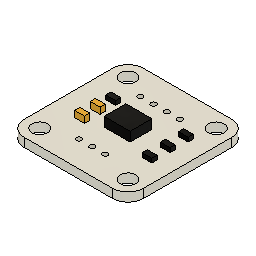
MambaMouse_Rev2 v16 (Autodesk Fusion 360 archive; units mm, degrees)
design "AS5600"
Autodesk Fusion 360 part; units mm, degrees
sketch "Sketch2" plane through (0, 0, 0) normal (0, 1, 0) x (1, 0, 0)
  line L0 (-8.5, -11.5) -> (8.5, -11.5)
  line L1 (11.5, -8.5) -> (11.5, 8.5)
  line L2 (8.5, 11.5) -> (-8.5, 11.5)
  line L3 (-11.5, 8.5) -> (-11.5, -8.5)
  line L4 (-11.5, -11.5) -> (11.5, 11.5) construction
  line L5 (11.5, -11.5) -> (-11.5, 11.5) construction
  line L6 (-8.5, 8.5) -> (8.5, 8.5) construction
  line L7 (8.5, 8.5) -> (8.5, -8.5) construction
  line L8 (8.5, -8.5) -> (-8.5, -8.5) construction
  line L9 (-8.5, -8.5) -> (-8.5, 8.5) construction
  line L10 (-8.5, 8.5) -> (8.5, -8.5) construction
  line L11 (8.5, 8.5) -> (-8.5, -8.5) construction
  circle A0 centre (-8.5, 8.5) radius 1.5
  circle A1 centre (8.5, 8.5) radius 1.5
  circle A2 centre (8.5, -8.5) radius 1.5
  circle A3 centre (-8.5, -8.5) radius 1.5
  arc A4 (-8.5, 11.5) -> (-11.5, 8.5) centre (-8.5, 8.5) ccw
  arc A5 (11.5, 8.5) -> (8.5, 11.5) centre (8.5, 8.5) ccw
  arc A6 (8.5, -11.5) -> (11.5, -8.5) centre (8.5, -8.5) ccw
  arc A7 (-11.5, -8.5) -> (-8.5, -11.5) centre (-8.5, -8.5) ccw
  line L12 (-2.5, -2.1) -> (2.5, -2.1)
  line L13 (2.5, -2.1) -> (2.5, 2.1)
  line L14 (2.5, 2.1) -> (-2.5, 2.1)
  line L15 (-2.5, 2.1) -> (-2.5, -2.1)
  line L16 (-2.5, -2.1) -> (2.5, 2.1) construction
  line L17 (2.5, -2.1) -> (-2.5, 2.1) construction
  circle A8 centre (-4.12, 6.5) radius 0.5
  circle A9 centre (-1.58, 6.5) radius 0.5
  circle A10 centre (0.96, 6.5) radius 0.5
  circle A11 centre (3.5, 6.5) radius 0.5
  line L18 (-4.12, 6.5) -> (-1.58, 6.5) construction
  line L19 (-1.58, 6.5) -> (0.96, 6.5) construction
  line L20 (0.96, 6.5) -> (3.5, 6.5) construction
  circle A12 centre (2.14, -6.5) radius 0.5
  circle A13 centre (-0.4, -6.5) radius 0.5
  circle A14 centre (-2.94, -6.5) radius 0.5
  line L21 (-2.94, -6.5) -> (-0.4, -6.5) construction
  line L22 (-0.4, -6.5) -> (2.14, -6.5) construction
  line L23 (-6.9, 3.63) -> (-5.02, 3.63)
  line L24 (-5.02, 3.63) -> (-5.02, 2.63)
  line L25 (-5.02, 2.63) -> (-6.9, 2.63)
  line L26 (-6.9, 2.63) -> (-6.9, 3.63)
  line L27 (-6.9, 0.63) -> (-5.02, 0.63)
  line L28 (-5.02, 0.63) -> (-5.02, -0.37)
  line L29 (-5.02, -0.37) -> (-6.9, -0.37)
  line L30 (-6.9, -0.37) -> (-6.9, 0.63)
  line L31 (-6.9, -2.37) -> (-5.02, -2.37)
  line L32 (-5.02, -2.37) -> (-5.02, -3.37)
  line L33 (-5.02, -3.37) -> (-6.9, -3.37)
  line L34 (-6.9, -3.37) -> (-6.9, -2.37)
  line L35 (-6.9, 2.63) -> (-6.9, 0.63) construction
  line L36 (-6.9, -0.37) -> (-6.9, -2.37) construction
  line L37 (6.22, 4.5) -> (8.1, 4.5)
  line L38 (8.1, 4.5) -> (8.1, 3.5)
  line L39 (8.1, 3.5) -> (6.22, 3.5)
  line L40 (6.22, 3.5) -> (6.22, 4.5)
  line L41 (6.22, 1) -> (8.1, 1)
  line L42 (8.1, 1) -> (8.1, 0)
  line L43 (8.1, 0) -> (6.22, 0)
  line L44 (6.22, 0) -> (6.22, 1)
  line L45 (6.22, -2.5) -> (8.1, -2.5)
  line L46 (8.1, -2.5) -> (8.1, -3.5)
  line L47 (8.1, -3.5) -> (6.22, -3.5)
  line L48 (6.22, -3.5) -> (6.22, -2.5)
  line L49 (8.1, -2.5) -> (8.1, 0) construction
  line L50 (8.1, 3.5) -> (8.1, 1) construction
  dimension "d6" = 23
  dimension "d7" = 23
  dimension "d8" = 17
  dimension "d9" = 17
  dimension "d10" = 3
  dimension "d11" = 3
  dimension "d12" = 3
  dimension "d13" = 3
  dimension "d14" = 3
  dimension "d15" = 5
  dimension "d16" = 4.2
  dimension "d21" = 1
  dimension "d25" = 2.54
  dimension "d26" = 2.54
  dimension "d27" = 2.54
  dimension "d28" = 5
  dimension "d29" = 8
  dimension "d30" = 2.54
  dimension "d31" = 2.54
  dimension "d32" = 5
  dimension "d33" = 8.56
  dimension "d34" = 1.88
  dimension "d35" = 1
  dimension "d36" = 2
  dimension "d37" = 2
  dimension "d38" = 4.6
  dimension "d39" = 8.13
  dimension "d41" = 3.4
  dimension "d42" = 2.5
  dimension "d43" = 2.5
  dimension "d44" = 8
  constraint horizontal L0
  constraint perpendicular L0 L1
  constraint parallel L0 L2
  constraint parallel L1 L3
  constraint coincident L4 origin
  constraint coincident L5 origin
  constraint horizontal L6
  constraint perpendicular L6 L7
  constraint parallel L6 L8
  constraint parallel L7 L9
  constraint coincident L10 origin
  constraint coincident L11 origin
  constraint coincident L6.start L9.end
  constraint coincident L6.end L7.start
  constraint coincident L7.end L8.start
  constraint coincident L8.end L9.start
  constraint equal A0 A3
  constraint equal A1 A3
  constraint equal A2 A3
  constraint coincident L5.end L3
  constraint coincident L5.end L2
  constraint tangent L3 A4
  constraint tangent L2 A4
  constraint coincident L4.end L2
  constraint coincident L4.end L1
  constraint tangent L2 A5
  constraint tangent L1 A5
  constraint coincident L5.start L0
  constraint coincident L5.start L1
  constraint tangent L0 A6
  constraint tangent L1 A6
  constraint coincident L4.start L3
  constraint coincident L4.start L0
  constraint tangent L3 A7
  constraint tangent L0 A7
  constraint horizontal L12
  constraint perpendicular L12 L13
  constraint parallel L12 L14
  constraint parallel L13 L15
  constraint coincident L16 origin
  constraint coincident L17 origin
  constraint coincident A8.centre L18.start
  constraint coincident A9.centre L18.end
  constraint parallel L6 L18
  constraint coincident A10.centre L19.end
  constraint coincident A11.centre L20.end
  constraint horizontal L19
  constraint horizontal L20
  constraint equal A8 A9
  constraint equal A8 A10
  constraint equal A8 A11
  constraint equal A8 A14
  constraint equal A9 A13
  constraint equal A10 A12
  constraint coincident A14.centre L21.start
  constraint coincident A13.centre L21.end
  constraint horizontal L21
  constraint coincident A12.centre L22.end
  constraint horizontal L22
  constraint horizontal L23
  constraint vertical L24
  constraint horizontal L25
  constraint vertical L26
  constraint horizontal L27
  constraint vertical L28
  constraint horizontal L29
  constraint vertical L30
  constraint horizontal L31
  constraint vertical L32
  constraint horizontal L33
  constraint vertical L34
  constraint equal L23 L27
  constraint equal L27 L31
  constraint equal L24 L28
  constraint equal L28 L32
  constraint vertical L35
  constraint vertical L36
  constraint horizontal L37
  constraint vertical L38
  constraint horizontal L39
  constraint vertical L40
  constraint horizontal L41
  constraint vertical L42
  constraint horizontal L43
  constraint vertical L44
  constraint horizontal L45
  constraint vertical L46
  constraint horizontal L47
  constraint vertical L48
  constraint equal L23 L37
  constraint equal L24 L38
  constraint equal L23 L41
  constraint equal L24 L42
  constraint equal L23 L45
  constraint equal L24 L48
  constraint vertical L50
  constraint vertical L49
  measures "d6" distance of L4.start L5.start
  measures "d7" distance of L5.start L4.end
  measures "d8" distance of L7.end L8.end
  measures "d9" distance of L6.end L7.end
  measures "d10" diameter of A3
  measures "d11" radius of A4
  measures "d12" radius of A5
  measures "d13" radius of A6
  measures "d14" radius of A7
  measures "d15" distance of L13.end L14.end
  measures "d16" distance of L12.end L13.end
  measures "d21" diameter of A8
  measures "d25" distance of A8.centre A9.centre
  measures "d26" horizontal distance of A9.centre A10.centre
  measures "d27" horizontal distance of A10.centre A11.centre
  measures "d28" distance of L2 L18
  measures "d29" distance of L1 A11.centre
  measures "d30" distance of A13.centre A14.centre
  measures "d31" horizontal distance of A12.centre A13.centre
  measures "d32" distance of L0 L22
  measures "d33" distance of L3 A14.centre
  measures "d34" distance of L23.start L23.end
  measures "d35" distance of L23.end L24.end
  measures "d36" distance of L25 L27
  measures "d37" distance of L29 L31
  measures "d38" distance of L3 L35
  measures "d39" distance of L0 L33
  measures "d41" distance of L1 L50
  measures "d42" distance of L38.end L41.end
  measures "d43" distance of L42.end L45.end
  measures "d44" distance of L0 L47
extrude "Extrude1" add sketch "Sketch2" against normal blind 1.7 contours L0 L1 L2 L3 A4 A5 A6 A7 | L12 L13 L14 L15 | L23 L24 L25 L26 | L27 L28 L29 L30 | L31 L32 L33 L34 | L37 L38 L39 L40 | L41 L42 L43 L44 | L45 L46 L47 L48
extrude "Extrude2" add sketch "Sketch2" along normal blind 1.8 contours L12 L13 L14 L15
extrude "Extrude3" add sketch "Sketch2" along normal blind 0.8 contours L23 L24 L25 L26 | L37 L38 L39 L40 | L41 L42 L43 L44 | L45 L46 L47 L48
extrude "Extrude4" add sketch "Sketch2" along normal blind 1.22 contours L27 L28 L29 L30 | L31 L32 L33 L34
